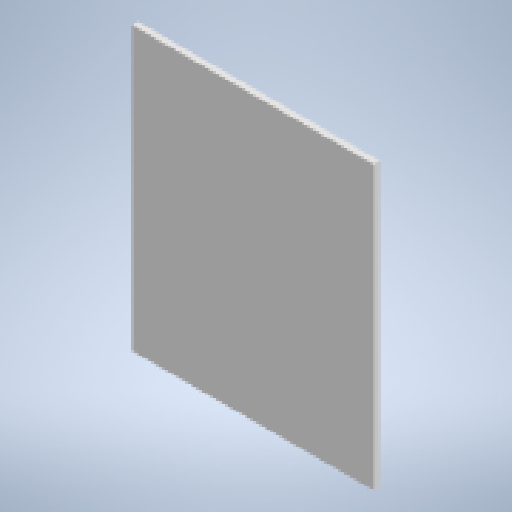
# Autodesk Inventor part: плата верные раземры
Saved by Autodesk Inventor 2024.2 (Build 282272000, 272)
## iProperties
Created: 2026-04-24
Part Number: плата верные раземры
Material: Типовые
Document SubType Name: Modeling
Designer: katya_notebook
Density: 1 g/cm^3
Appearance: По умолчанию
Author: katya_notebook
Autodesk Inventor part; units mm, degrees
ref_plane "YZ Plane" through (0, 0, 0) normal (1, 0, 0) x (0, 1, 0)
ref_plane "XZ Plane" through (0, 0, 0) normal (0, 1, 0) x (-1, 0, 0)
ref_plane "XY Plane" through (0, 0, 0) normal (0, 0, 1) x (1, 0, 0)
ref_plane "РабПлоскость1" through (0, 0, 0) normal (0, 0, 1) x (1, 0, 0)
sketch "Эскиз1" plane through (0, 0, 0) normal (0, 0, 1) x (1, 0, 0)
  line L0 (0.77, 24.63) -> (1.77, 24.63) projected
  line L1 (1.77, 24.63) -> (1.77, 23.63) projected
  line L2 (1.77, 23.63) -> (0.77, 23.63) projected
  line L3 (0.77, 23.63) -> (0.77, 24.63) projected
  circle A0 centre (1.27, 24.13) radius 0.0769
  line L4 (4.27, 38.13) -> (-55.73, 38.13)
  line L5 (-55.73, 38.13) -> (-55.73, -31.87)
  line L6 (-55.73, -31.87) -> (4.27, -31.87)
  line L7 (4.27, -31.87) -> (4.27, 38.13)
  line L8 (0.77, 23.63) -> (1.77, 24.63)
  line L9 (0.77, 24.63) -> (1.77, 23.63)
  point P0 (0, 0)
  point P1 (1.27, 24.13)
  point P2 (1.27, 24.13)
  dimension "d0" = 3
  dimension "d1" = 70
  dimension "d2" = 60
  dimension "d3" = 14
  constraints: 12 end point, 2 midpoint, 2 parallel, 2 perpendicular, 1 centre point, 1 coincident, 1 horizontal
  measures "d0" distance from line of L7 A0.centre
  measures "d1" distance of L6.end L4.start
  measures "d2" distance of L5.end L6.end
  measures "d3" distance from line of L4 point (1.27, 24.13)
extrude "Выдавливание1" add sketch "Эскиз1" along normal blind 1.5 contours L9 A0 L8 L3 | L0 L8 A0 L9 | L1 L9 A0 L8 | L8 A0 L9 L2 | L9 L8 A0 | A0 L8 L9 | A0 L9 L8 | L8 L9 A0 | L7 L6 L5 L4
